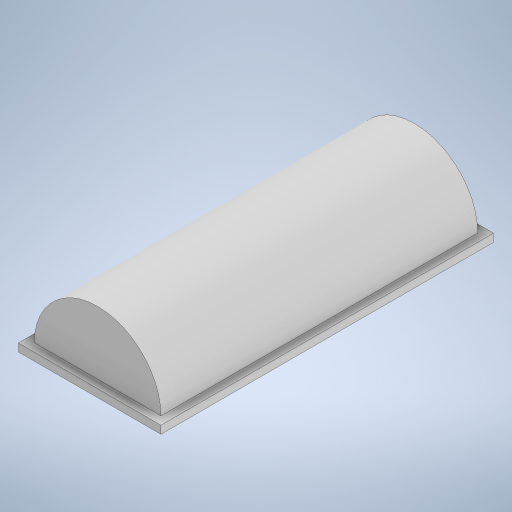
# Autodesk Inventor part: Project
Saved by Autodesk Inventor 2023.3 (Build 273359000, 359)
## iProperties
Created: 2023-12-02
Part Number: Project
Material: Generic
Document SubType Name: Modeling
Designer: Oasis
Density: 1 g/cm^3
Appearance: Default
Author: Oasis
Autodesk Inventor part; units mm, degrees
ref_plane "YZ Plane" through (0, 0, 0) normal (1, 0, 0) x (0, 1, 0)
ref_plane "XZ Plane" through (0, 0, 0) normal (0, 1, 0) x (-1, 0, 0)
ref_plane "XY Plane" through (0, 0, 0) normal (0, 0, 1) x (1, 0, 0)
sketch "Sketch1" plane through (0, 0, 0) normal (0, 0, 1) x (1, 0, 0)
  line L0 (0, 0) -> (40, 0)
  arc A0 (40, 0) -> (-40, 0) centre (0, 0) ccw
  line L1 (0, 0) -> (-40, 0)
  line L2 (0, 5) -> (34.641, 5)
  arc A1 (34.641, 5) -> (-34.641, 5) centre (0, 0) ccw
  line L3 (-34.641, 5) -> (0, 5)
  line L4 (40, 0) -> (45, 0)
  line L5 (45, 0) -> (45, -5)
  line L6 (45, -5) -> (-45, -5)
  line L7 (-45, -5) -> (-45, 0)
  line L8 (-45, 0) -> (-40, 0)
  dimension "d0" = 40
  dimension "d1" = 5
  dimension "d2" = 5
  dimension "d3" = 5
  dimension "d4" = 90
  constraints: 18 end point, 4 perpendicular, 4 point on circle, 3 horizontal, 2 centre point, 1 coincident, 1 point on line, 2 other
  measures "d0" distance of L0.start L0.end
  measures "d1" distance between parallel lines of L0 L2
  measures "d2" distance of L0.end L4.end
  measures "d3" distance of L4.end L5.end
  measures "d4" distance of L5.end L6.end
extrude "Extrusion1" add sketch "Sketch1" along normal mid plane 190 contours L3 A1 L2
extrude "Extrusion2" add sketch "Sketch1" along normal mid plane 200 separate body contours L1 A0 L0
extrude "Extrusion3" add sketch "Sketch1" along normal mid plane 210 separate body contours L0 L4 L5 L6 L7 L8 L1
sketch "Sketch2" plane through (0, 0, 100) normal (0, 0, 1) x (1, 0, 0)
  arc A0 (34.641, 5) -> (-34.641, 5) centre (0, 0) ccw projected
  line L0 (34.641, 5) -> (-34.641, 5) projected
extrude "Extrusion4" add sketch "Sketch2" against normal blind 5 separate body
sketch "Sketch3" plane through (0, 0, -100) normal (0, 0, -1) x (-1, 0, 0)
  arc A0 (34.641, 5) -> (-34.641, 5) centre (0, 0) ccw projected
  line L0 (34.641, 5) -> (-34.641, 5) projected
extrude "Extrusion5" add sketch "Sketch3" against normal blind 5 separate body
combine bodies "Combine1" operation type add bodies to combine 5 4 2
body "Solid1"
body "Solid2"
body "Solid3"
